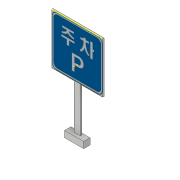
# Autodesk Inventor part: parkinglot
Saved by Autodesk Inventor 2018 (Build 220112000, 112)
## iProperties
Created: 2017-08-24
Part Number: parkinglot
Material: Generic
Document SubType Name: Modeling
Designer: Platform
Density: 1 g/cm^3
Appearance: Default
Author: Platform
Autodesk Inventor part; units mm, degrees
ref_plane "YZ Plane" through (0, 0, 0) normal (1, 0, 0) x (0, 1, 0)
ref_plane "XZ Plane" through (0, 0, 0) normal (0, 1, 0) x (-1, 0, 0)
ref_plane "XY Plane" through (0, 0, 0) normal (0, 0, 1) x (1, 0, 0)
sketch "Sketch1" plane through (0, 0, 0) normal (0, 0, 1) x (1, 0, 0)
  line L0 (-40, 55.2261) -> (40, 55.2261)
  line L1 (40, 55.2261) -> (40, -24.3415)
  line L2 (40, -24.3415) -> (-40, -24.3415)
  line L3 (-40, -24.3415) -> (-40, 55.2261)
  point P0 (0, 0)
  dimension "d8" = 24.3415
  constraints: 8 end point, 2 parallel, 1 horizontal, 1 perpendicular
  measures "d8" vertical distance of L1.end point (0, 0)
extrude "Extrusion1" add sketch "Sketch1" against normal blind 2
sketch "Sketch2" plane through (0, 0, 0) normal (0, 0, 1) x (1, 0, 0)
  line L0 (-40, 55.2261) -> (40, 55.2261) projected
  line L1 (-40, 55.2261) -> (39.9042, 55.2261) construction
  line L2 (39.9042, 55.2261) -> (39.9042, -24.6781) construction
  line L3 (39.9042, -24.6781) -> (-40, -24.6781) construction
  line L4 (-40, -24.6781) -> (-40, 55.2261) construction
  point P0 (0, 0)
  constraints: 2 other
sketch "Sketch3" plane through (0, 0, 0) normal (0, 0, 1) x (1, 0, 0)
  line L0 (40, -24.3415) -> (-40, -24.3415) projected
  line L1 (-5, -24.3415) -> (5, -24.3415)
  line L2 (5, -24.3415) -> (5, -94.3415)
  line L3 (5, -94.3415) -> (-5, -94.3415)
  line L4 (-5, -94.3415) -> (-5, -24.3415)
  line L5 (-15, -94.3415) -> (15, -94.3415)
  line L6 (15, -94.3415) -> (15, -104.3415)
  line L7 (15, -104.3415) -> (-15, -104.3415)
  line L8 (-15, -104.3415) -> (-15, -94.3415)
  point P0 (0, 0)
  dimension "d12" = 10
  dimension "d13" = 70
  dimension "d14" = 5
  dimension "d15" = 30
  dimension "d16" = 10
  constraints: 16 end point, 4 parallel, 2 horizontal, 2 perpendicular, 1 point on line
  measures "d12" distance of L2.end L3.end
  measures "d13" distance of L1.end L2.end
  measures "d14" horizontal distance of point (0, 0) L1.end
  measures "d15" distance of L6.end L7.end
  measures "d16" distance of L5.end L6.end
extrude "Extrusion2" add sketch "Sketch3" along normal mid plane 10 contours L5 L6 L7 L8 L3
sketch "Sketch4" plane through (0, 0, 5) normal (0, 0, 1) x (1, 0, 0)
  point P0 (0, 0)
sketch "Sketch7" plane through (0, 0, -2) normal (0, 0, -1) x (-1, 0, 0)
  line L0 (-40, -24.3415) -> (40, -24.3415) projected
  line L1 (-15, -94.3415) -> (15, -94.3415) projected
  line L2 (-4.9075, -24.3415) -> (5.0925, -24.3415)
  line L3 (5.0925, -24.3415) -> (5.0925, -94.3415)
  line L4 (5.0925, -94.3415) -> (-4.9075, -94.3415)
  line L5 (-4.9075, -94.3415) -> (-4.9075, -24.3415)
  point P0 (0, 0)
  dimension "d21" = 10
  constraints: 8 end point, 2 parallel, 2 point on line, 1 horizontal, 1 perpendicular
  measures "d21" distance between parallel lines of L5 L3
extrude "Extrusion3" add sketch "Sketch7" against normal blind 2
body "Solid1"
